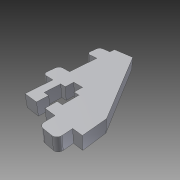
# Autodesk Inventor part: x_carryage_brace
Saved by Autodesk Inventor 2014 (Build 180170000, 170)
## iProperties
Created: 2013-11-07
Part Number: x_carryage_brace
Material: Aluminum 6061
Document SubType Name: Modeling
Designer: buben
Density: 1 g/cm^3
Appearance: Aluminum - Flat
Author: buben
Subject: Laser Cutted
Autodesk Inventor part; units mm, degrees
ref_plane "YZ Plane" through (0, 0, 0) normal (1, 0, 0) x (0, 1, 0)
ref_plane "XZ Plane" through (0, 0, 0) normal (0, 1, 0) x (-1, 0, 0)
ref_plane "XY Plane" through (0, 0, 0) normal (0, 0, 1) x (1, 0, 0)
sketch "Sketch1" plane through (0, 0, 0) normal (0, 0, 1) x (1, 0, 0)
  line L0 (0, 46) -> (0, 0)
  line L1 (0, 0) -> (28, 0)
  line L2 (28, 0) -> (28, 10)
  line L3 (0, 46) -> (10, 46)
  line L4 (10, 46) -> (28, 10)
  dimension "d0" = 10
  dimension "d1" = 10
  dimension "d2" = 46
  dimension "d3" = 28
  constraints: 10 end point, 2 perpendicular, 1 parallel, 1 vertical
  measures "d0" distance of L0.start L3.end
  measures "d1" distance of L1.end L2.end
  measures "d2" distance of L0.start L0.end
  measures "d3" distance of L0.end L1.end
extrude "Extrusion1" add sketch "Sketch1" along normal blind 6
sketch "Sketch2" plane through (0, 0, 6) normal (0, 0, 1) x (1, 0, 0)
  line L0 (0, 46) -> (0, 0) projected
  line L1 (0, 0) -> (28, 0) projected
  line L2 (0, 43) -> (-4, 43)
  line L3 (-6, 41) -> (-6, 37)
  line L4 (-4, 35) -> (0, 35)
  line L5 (0, 35) -> (0, 43)
  line L6 (0, 20) -> (-4, 20)
  line L7 (-6, 18) -> (-6, 14)
  line L8 (-4, 12) -> (0, 12)
  line L9 (0, 12) -> (0, 20)
  line L10 (16, 0) -> (24, 0)
  line L11 (24, 0) -> (24, -4)
  line L12 (22, -6) -> (18, -6)
  line L13 (16, -4) -> (16, 0)
  arc A0 (-4, 43) -> (-6, 41) centre (-4, 41) ccw
  arc A1 (-6, 37) -> (-4, 35) centre (-4, 37) ccw
  arc A2 (-4, 20) -> (-6, 18) centre (-4, 18) ccw
  arc A3 (-6, 14) -> (-4, 12) centre (-4, 14) ccw
  arc A4 (16, -4) -> (18, -6) centre (18, -4) ccw
  arc A5 (22, -6) -> (24, -4) centre (22, -4) ccw
  line L14 (28, 0) -> (28, 10) projected
  point P0 (-6, 35)
  point P1 (-6, 43)
  point P2 (-6, 12)
  point P3 (-6, 20)
  point P4 (24, -6)
  point P5 (16, -6)
  dimension "d6" = 8
  dimension "d7" = 8
  dimension "d9" = 8
  dimension "d10" = 12
  dimension "d11" = 15
  dimension "d15" = 2
  dimension "d16" = 6
  dimension "d38" = 4
  dimension "d39" = 6
  constraints: 24 end point, 15 point on line, 12 point on circle, 12 tangent, 6 centre point, 6 parallel, 5 equal radius, 3 horizontal, 3 perpendicular, 1 collinear
  measures "d6" distance of point (-6, 20) point (-6, 12)
  measures "d7" distance of point (-6, 43) point (-6, 35)
  measures "d9" distance of point (24, -6) point (16, -6)
  measures "d10" distance from line of L0.end L8
  measures "d11" distance between parallel lines of L4 L6
  measures "d15" radius of A0
  measures "d16" distance between parallel lines of L0 L3
  measures "d38" distance between parallel lines of L14 L11
  measures "d39" distance between parallel lines of L1 L12
sketch "Sketch3" plane through (0, 0, 6) normal (0, 0, 1) x (1, 0, 0)
  line L0 (0, 0) -> (28, 0) projected
  line L1 (6.5, 0) -> (6.5, 5)
  line L2 (6.5, 5) -> (4, 5)
  line L3 (4, 5) -> (4, 12.3)
  line L4 (4, 12.3) -> (6.5, 12.3)
  line L5 (6.5, 12.3) -> (6.5, 16.3)
  line L6 (6.5, 16.3) -> (11, 16.3)
  line L7 (11, 16.3) -> (11, 12.3)
  line L8 (11, 12.3) -> (13.5, 12.3)
  line L9 (13.5, 12.3) -> (13.5, 5)
  line L10 (13.5, 5) -> (11, 5)
  line L11 (11, 5) -> (11, 0)
  line L12 (0, 46) -> (0, 0) projected
  point P0 (11, 0)
  point P1 (26, 0)
  point P2 (8.75, 16.3)
  dimension "d27" = 4.5
  dimension "d28" = 5
  dimension "d29" = 7.3
  dimension "d30" = 4
  dimension "d32" = 2.5
  dimension "d33" = 2.5
  dimension "d41" = 4
  constraints: 22 end point, 6 collinear, 6 parallel, 2 perpendicular, 2 point on line, 1 midpoint
  measures "d27" distance of L5.end L6.end
  measures "d28" distance of L1.start L1.end
  measures "d29" distance of L2.end L3.end
  measures "d30" distance of L4.end L5.end
  measures "d32" distance of L3.end L4.end
  measures "d33" distance of L7.end L8.end
  measures "d41" distance between parallel lines of L12 L3
extrude "Extrusion4" cut sketch "Sketch3" against normal through all
extrude "Extrusion5" add sketch "Sketch2" against normal blind 6
body "Solid1"
